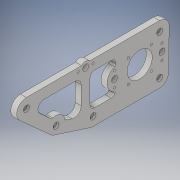
# Autodesk Inventor part: Frame_Stepper_New
Saved by Autodesk Inventor 2019 (Build 230136000, 136)
## iProperties
Created: 2019-10-21
Part Number: Frame_Stepper_New
Material: Generic
Document SubType Name: Modeling
Designer: 19879326
Density: 1 g/cm^3
Appearance: Default
Author: 19879326
Autodesk Inventor part; units mm, degrees
ref_plane "YZ Plane" through (0, 0, 0) normal (1, 0, 0) x (0, 1, 0)
ref_plane "XZ Plane" through (0, 0, 0) normal (0, 1, 0) x (-1, 0, 0)
ref_plane "XY Plane" through (0, 0, 0) normal (0, 0, 1) x (1, 0, 0)
sketch "Sketch1" plane through (0, 0, 0) normal (1, 0, 0) x (0, 1, 0)
  circle A0 centre (33, 0) radius 4
  circle A1 centre (-29, -10) radius 4
  circle A2 centre (-29, -100) radius 4
  circle A3 centre (25, 80) radius 4
  circle A4 centre (25, -100) radius 4
  arc A5 (38, -5.5902) -> (38, 5.5902) centre (33, 0) ccw
  line L0 (38, -5.5902) -> (38, -100)
  line L1 (38, 5.5902) -> (38, 80)
  arc A6 (38, 80) -> (15.333, 88.692) centre (25, 80) ccw
  arc A7 (24.7593, -112.9978) -> (38, -100) centre (25, -100) ccw
  circle A8 centre (0, -39) radius 4
  circle A9 centre (0, -73.15) radius 17
  circle A10 centre (15.5, -57.65) radius 1.5
  circle A11 centre (15.5, -88.65) radius 1.5
  circle A12 centre (-15.5, -57.65) radius 1.5
  circle A13 centre (-15.5, -88.65) radius 1.5
  circle A14 centre (-15, 40) radius 4
  line L2 (-41, -10) -> (-41, -100)
  arc A15 (-41, -100) -> (-29.2222, -111.9979) centre (-29, -100) ccw
  arc A16 (-40.4224, -6.3217) -> (-41, -10) centre (-29, -10) ccw
  line L3 (24.7593, -112.9978) -> (-29.2222, -111.9979)
  arc A17 (-14.6604, 28.0048) -> (-4.4611, 45.7386) centre (-15, 40) ccw
  line L4 (-4.4611, 45.7386) -> (9.9167, 61.7291)
  line L5 (24, 56.3287) -> (24, 14.0771)
  line L6 (-8.8485, 6) -> (15.9229, 6)
  arc A18 (24, 56.3287) -> (9.9167, 61.7291) centre (15.9229, 56.3287) ccw
  arc A19 (15.9229, 6) -> (24, 14.0771) centre (15.9229, 14.0771) ccw
  arc A20 (-17.793, 18.2771) -> (-8.8485, 6) centre (-8.8485, 15.3968) ccw
  line L7 (-17.793, 18.2771) -> (-14.6604, 28.0048)
  line L8 (19.5175, -6) -> (-14, -6)
  arc A21 (24, -12) -> (18, -6) centre (18, -12) ccw
  arc A22 (18, -40.65) -> (24, -34.65) centre (18, -34.65) ccw
  arc A23 (-14, -6) -> (-20, -12) centre (-14, -12) ccw
  arc A24 (-20, -34.65) -> (-15, -40.5661) centre (-14, -34.65) ccw
  line L9 (24, -12) -> (24, -34.65)
  line L10 (-20, -34.65) -> (-20, -12)
  line L11 (18, -40.65) -> (15, -40.65)
  arc A25 (15, -40.65) -> (-15, -40.5661) centre (-0.0109, -44.4957) ccw
  circle A26 centre (0, -103.15) radius 4
  circle A27 centre (10, -103.15) radius 1.5
  circle A28 centre (-10, -103.15) radius 1.5
  line L12 (15.333, 88.692) -> (-22.4361, 46.6861)
  line L13 (-40.4224, -6.3217) -> (-24.5186, 43.0652)
  arc A29 (-22.4361, 46.6861) -> (-24.5186, 43.0652) centre (-15, 40) ccw
  arc A30 (-14.6604, 28.0048) -> (-4.4611, 45.7386) centre (-15, 40) ccw
  point P0 (0, 0)
  point P1 (38, 41.5104)
  point P2 (38, -62.1387)
  point P3 (-20, -40.65)
  point P4 (16.5, -40.65)
  point P5 (-18, -40.65)
  point P6 (0, -29)
  point P7 (-10, -94.936)
  dimension "d0" = 8
  dimension "d1" = 8
  dimension "d2" = 8
  dimension "d3" = 8
  dimension "d4" = 80
  dimension "d5" = 100
  dimension "d6" = 62
  dimension "d7" = 90
  dimension "d8" = 10
  dimension "d9" = 15
  dimension "d10" = 5
  dimension "d13" = 8
  dimension "d14" = 39
  dimension "d15" = 34
  dimension "d16" = 34.15
  dimension "d17" = 3
  dimension "d18" = 3
  dimension "d19" = 3
  dimension "d20" = 3
  dimension "d21" = 31
  dimension "d22" = 31
  dimension "d23" = 15.5
  dimension "d24" = 15.5
  dimension "d25" = 8
  dimension "d27" = 12
  dimension "d28" = 24
  dimension "d29" = 24
  dimension "d30" = 24
  dimension "d31" = 33
  dimension "d34" = 14
  dimension "d35" = 6
  dimension "d38" = 6
  dimension "d42" = 6
  dimension "d46" = 9
  dimension "d47" = 14
  dimension "d48" = 17
  dimension "d97" = 15
  dimension "d98" = 10
  dimension "d110" = 15
  dimension "d117" = 8
  dimension "d118" = 30
  dimension "d121" = 3
  dimension "d122" = 3
  dimension "d123" = 10
  dimension "d124" = 10
  dimension "d134" = 40
  dimension "d135" = 15
  dimension "d136" = 42.2516
  dimension "d137" = 24.8066
  dimension "d139" = 10
  dimension "d145" = 14
  dimension "d146" = 14
  constraints: 33 point on circle, 31 centre point, 28 end point, 18 tangent, 11 vertical alignment, 8 horizontal alignment, 7 coincident, 6 equal radius, 4 parallel, 4 point on line, 4 vertical, 2 horizontal, 1 midpoint
  measures "d0" diameter of A0
  measures "d1" horizontal distance of A0.centre A3.centre
  measures "d2" diameter of A3
  measures "d3" diameter of A4
  measures "d4" vertical distance of A0.centre A3.centre
  measures "d5" vertical distance of A4.centre A0.centre
  measures "d6" horizontal distance of A1.centre A0.centre
  measures "d7" distance of A2.centre A1.centre
  measures "d8" vertical distance of A1.centre A0.centre
  measures "d9" diameter of A5
  measures "d10" distance from line of L0 A0.centre
  measures "d13" diameter of A8
  measures "d14" distance of A8.centre point (0, 0)
  measures "d15" diameter of A9
  measures "d16" distance of A8.centre A9.centre
  measures "d17" diameter of A10
  measures "d18" diameter of A11
  measures "d19" diameter of A12
  measures "d20" diameter of A13
  measures "d21" distance of A11.centre A10.centre
  measures "d22" distance of A10.centre A12.centre
  measures "d23" horizontal distance of A9.centre A10.centre
  measures "d24" horizontal distance of A9.centre A10.centre
  measures "d25" diameter of A14
  measures "d27" distance from line of L2 A1.centre
  measures "d28" diameter of A15
  measures "d29" diameter of A16
  measures "d30" diameter of A17
  measures "d31" distance of A0.centre point (0, 0)
  measures "d34" distance between parallel lines of L1 L5
  measures "d35" distance from line of point (0, 0) L6
  measures "d38" distance from line of point (0, 0) L8
  measures "d42" radius of A21
  measures "d46" distance from line of A1.centre L10
  measures "d47" distance between parallel lines of L0 L9
  measures "d48" distance from line of A10.centre L11
  measures "d97" horizontal distance of L11.end A8.centre
  measures "d98" distance of point (0, -29) A8.centre
  measures "d110" horizontal distance of A8.centre A24.end
  measures "d117" diameter of A26
  measures "d118" distance of A9.centre A26.centre
  measures "d121" diameter of A27
  measures "d122" diameter of A28
  measures "d123" distance of A26.centre A27.centre
  measures "d124" distance of A28.centre A26.centre
  measures "d134" vertical distance of A17.centre point (0, 0)
  measures "d135" horizontal distance of point (0, 0) A14.centre
  measures "d136" distance of A18.centre A19.centre
  measures "d137" distance of A19.centre A20.centre
  measures "d139" radius of A29
  measures "d145" distance between parallel lines of L12 L4
  measures "d146" distance between parallel lines of L13 L7
extrude "Extrusion1" add sketch "Sketch1" along normal blind 8
sketch "Sketch3" plane through (0, 0, 0) normal (-1, 0, 0) x (0, 0, 1)
  circle A0 centre (-100, 25) radius 4 projected
  line L0 (-92.4944, 25) -> (-96.2472, 18.5)
  line L1 (-96.2472, 18.5) -> (-103.7528, 18.5)
  line L2 (-103.7528, 18.5) -> (-107.5056, 25)
  line L3 (-107.5056, 25) -> (-103.7528, 31.5)
  line L4 (-103.7528, 31.5) -> (-96.2472, 31.5)
  line L5 (-96.2472, 31.5) -> (-92.4944, 25)
  line L6 (-100, 38) -> (-5.5902, 38) projected
  circle A1 centre (-100, -29) radius 4 projected
  line L7 (-96.2472, -22.5) -> (-92.4944, -29)
  line L8 (-92.4944, -29) -> (-96.2472, -35.5)
  line L9 (-96.2472, -35.5) -> (-103.7528, -35.5)
  line L10 (-103.7528, -35.5) -> (-107.5056, -29)
  line L11 (-107.5056, -29) -> (-103.7528, -22.5)
  line L12 (-103.7528, -22.5) -> (-96.2472, -22.5)
  circle A2 centre (40, -15) radius 4 projected
  line L13 (47.5056, -15) -> (43.7528, -21.5)
  line L14 (43.7528, -21.5) -> (36.2472, -21.5)
  line L15 (36.2472, -21.5) -> (32.4944, -15)
  line L16 (32.4944, -15) -> (36.2472, -8.5)
  line L17 (36.2472, -8.5) -> (43.7528, -8.5)
  line L18 (43.7528, -8.5) -> (47.5056, -15)
  circle A3 centre (-10, -29) radius 4 projected
  line L19 (-2.4944, -29) -> (-6.2472, -35.5)
  line L20 (-6.2472, -35.5) -> (-13.7528, -35.5)
  line L21 (-13.7528, -35.5) -> (-17.5056, -29)
  line L22 (-17.5056, -29) -> (-13.7528, -22.5)
  line L23 (-13.7528, -22.5) -> (-6.2472, -22.5)
  line L24 (-6.2472, -22.5) -> (-2.4944, -29)
  circle A4 centre (80, 25) radius 4 projected
  line L25 (87.5056, 25) -> (83.7528, 18.5)
  line L26 (83.7528, 18.5) -> (76.2472, 18.5)
  line L27 (76.2472, 18.5) -> (72.4944, 25)
  line L28 (72.4944, 25) -> (76.2472, 31.5)
  line L29 (76.2472, 31.5) -> (83.7528, 31.5)
  line L30 (83.7528, 31.5) -> (87.5056, 25)
  point P0 (0, 0)
  dimension "d61" = 13
  dimension "d62" = 13
  dimension "d63" = 13
  dimension "d64" = 13
  dimension "d65" = 13
  constraints: 60 end point, 5 coincident, 5 parallel, 65 other
  measures "d61" distance between parallel lines of L1 L4
  measures "d62" distance between parallel lines of L9 L12
  measures "d63" distance between parallel lines of L20 L23
  measures "d64" distance between parallel lines of L14 L17
  measures "d65" distance between parallel lines of L26 L29
extrude "Extrusion2" cut sketch "Sketch3" against normal blind 5
fillet "Fillet2" radius 2.5 3 edges at (4, 15, -40.65) (4, -4.4611, 45.7386) (4, -14.6604, 28.0048)
sketch "Sketch5" plane through (0, 0, 0) normal (-1, 0, 0) x (0, 0, 1)
  arc A0 (-80, 35) -> (-80, 27) centre (-80, 31) ccw
  arc A1 (-20, 27) -> (-20, 35) centre (-20, 31) ccw
  arc A2 (20, 35) -> (20, 27) centre (20, 31) ccw
  arc A3 (60, 27) -> (60, 35) centre (60, 31) ccw
  line L0 (-80, 35) -> (-20, 35)
  line L1 (-20, 27) -> (-80, 27)
  line L2 (20, 27) -> (60, 27)
  line L3 (60, 35) -> (20, 35)
  line L4 (-100, 38) -> (-5.5902, 38) projected
  line L5 (5.5902, 38) -> (80, 38) projected
  circle A4 centre (-100, 25) radius 4 projected
  circle A5 centre (0, 33) radius 4 projected
  circle A6 centre (80, 25) radius 4 projected
  arc A7 (-99.7609, 12.0926) -> (-109.7592, 11.9074) centre (-104.7601, 12) ccw
  arc A8 (-109.2406, -16.0926) -> (-99.2423, -15.9074) centre (-104.2415, -16) ccw
  line L6 (-111.9979, -29.2222) -> (-112.9978, 24.7593) projected
  circle A9 centre (-100, -29) radius 4 projected
  arc A10 (-80, -30) -> (-80, -38) centre (-80, -34) ccw
  arc A11 (-30, -38) -> (-30, -30) centre (-30, -34) ccw
  line L7 (-80, -30) -> (-30, -30)
  line L8 (-30, -38) -> (-80, -38)
  line L9 (-10, -41) -> (-100, -41) projected
  circle A12 centre (-10, -29) radius 4 projected
  arc A13 (3.7739, -25.6151) -> (6.2261, -33.23) centre (5, -29.4225) ccw
  circle A14 centre (40, -15) radius 4 projected
  line L10 (3.7739, -25.6151) -> (23.4454, -19.2804)
  line L11 (34.0688, -24.264) -> (6.2261, -33.23)
  circle A15 centre (-103.15, 0) radius 4 projected
  line L12 (-99.7609, 12.0926) -> (-99.6492, 6.0617)
  line L13 (-99.4272, -5.9279) -> (-99.2423, -15.9074)
  line L14 (23.4454, -19.2804) -> (29.2663, -17.4059)
  arc A16 (-99.6492, 6.0617) -> (-109.5895, 2.7446) centre (-103.15, 0) ccw
  arc A17 (-109.4835, -2.9812) -> (-99.4272, -5.9279) centre (-103.15, 0) ccw
  line L15 (-109.2406, -16.0926) -> (-109.4835, -2.9812)
  line L16 (-109.5895, 2.7446) -> (-109.7592, 11.9074)
  line L17 (26.4363, -15.1655) -> (18.2771, -17.793) projected
  arc A18 (74.9657, 7.0256) -> (69.6168, 12.9744) centre (72.2912, 10) ccw
  line L18 (69.6168, 12.9744) -> (47.4772, -6.9321)
  line L19 (74.9657, 7.0256) -> (50.99, -14.5319)
  line L20 (61.7291, 9.9167) -> (46.9639, -3.3594) projected
  line L21 (43.0652, -24.5186) -> (-6.3217, -40.4224) projected
  line L22 (88.692, 15.333) -> (46.6861, -22.4361) projected
  arc A19 (50.99, -14.5319) -> (47.4772, -6.9321) centre (40, -15) ccw
  arc A20 (29.2663, -17.4059) -> (34.0688, -24.264) centre (40, -15) ccw
  arc A21 (29.2663, -17.4059) -> (34.0688, -24.264) centre (40, -15) ccw
  arc A22 (50.99, -14.5319) -> (47.4772, -6.9321) centre (40, -15) ccw
  point P0 (0, 0)
  dimension "d71" = 8
  dimension "d72" = 8
  dimension "d73" = 8
  dimension "d74" = 3
  dimension "d75" = 3
  dimension "d76" = 20
  dimension "d77" = 20
  dimension "d78" = 20
  dimension "d79" = 20
  dimension "d80" = 10
  dimension "d83" = 13
  dimension "d84" = 13
  dimension "d85" = 3
  dimension "d86" = 8
  dimension "d87" = 20
  dimension "d88" = 20
  dimension "d89" = 8
  dimension "d92" = 15
  dimension "d128" = 3
  dimension "d129" = 7
  dimension "d130" = 7
  dimension "d140" = 8
  dimension "d141" = 3
  dimension "d142" = 3
  dimension "d143" = 15
  dimension "d144" = 11
  constraints: 33 point on circle, 30 end point, 22 tangent, 16 centre point, 14 parallel, 3 coincident, 2 equal radius, 1 collinear, 1 point on line
  measures "d71" diameter of A1
  measures "d72" diameter of A2
  measures "d73" diameter of A3
  measures "d74" distance between parallel lines of L4 L0
  measures "d75" distance between parallel lines of L5 L3
  measures "d76" horizontal distance of A4.centre A0.centre
  measures "d77" horizontal distance of A5.centre A1.centre
  measures "d78" horizontal distance of A2.centre A5.centre
  measures "d79" horizontal distance of A6.centre A3.centre
  measures "d80" diameter of A7
  measures "d83" vertical distance of A4.centre A7.centre
  measures "d84" vertical distance of A9.centre A8.centre
  measures "d85" distance between parallel lines of L9 L8
  measures "d86" diameter of A11
  measures "d87" horizontal distance of A9.centre A10.centre
  measures "d88" horizontal distance of A12.centre A11.centre
  measures "d89" diameter of A13
  measures "d92" horizontal distance of A12.centre A13.centre
  measures "d128" distance between parallel lines of L6 L16
  measures "d129" radius of A16
  measures "d130" radius of A17
  measures "d140" diameter of A18
  measures "d141" distance between parallel lines of L21 L11
  measures "d142" distance between parallel lines of L22 L19
  measures "d143" vertical distance of A6.centre A18.centre
  measures "d144" radius of A22
extrude "Extrusion3" cut sketch "Sketch5" against normal blind 5 contours L0 A1 L1 A0 | L3 A3 L2 A2 | L12 A16 L16 A7 | L15 A17 L13 A8 | L7 A11 L8 A10 | L10 L14 A20 L11 A13 | L19 A19 L18 A18
sketch "Sketch6" plane through (0, 0, 0) normal (-1, 0, 0) x (0, 0, 1)
  circle A0 centre (-39, 10) radius 1.5
  circle A1 centre (-39, -10) radius 1.5
  circle A2 centre (-10, 33) radius 1.5
  circle A3 centre (10, 33) radius 1.5
  circle A4 centre (-39, 0) radius 4 projected
  circle A5 centre (0, 33) radius 4 projected
  point P0 (0, 0)
  dimension "d99" = 3
  dimension "d100" = 3
  dimension "d101" = 3
  dimension "d102" = 3
  dimension "d103" = 10
  dimension "d105" = 10
  dimension "d106" = 10
  dimension "d107" = 10
  constraints: 4 centre point, 2 horizontal alignment, 2 vertical alignment
  measures "d99" diameter of A0
  measures "d100" diameter of A1
  measures "d101" diameter of A2
  measures "d102" diameter of A3
  measures "d103" distance of A4.centre A0.centre
  measures "d105" distance of A4.centre A1.centre
  measures "d106" distance of A5.centre A2.centre
  measures "d107" distance of A5.centre A3.centre
extrude "Extrusion4" cut sketch "Sketch6" against normal blind 10 contours A0 | A1 | A2 | A3
fillet "Fillet3" radius 2 1 edges at (4, -15, -40.5661)
fillet "Fillet4" radius 2 2 edges at (2.5, 2.7446, -109.5895) (2.5, -2.9812, -109.4835)
fillet "Fillet5" radius 1 6 edges at (2.5, 6.0617, -99.6492) (2.5, -5.9279, -99.4272) (2.5, -17.4059, 29.2663) (2.5, -24.264, 34.0688) (2.5, -6.9321, 47.4772) (2.5, -14.5319, 50.99)
body "Solid1"
